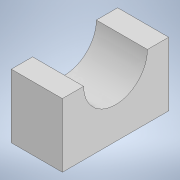
# Autodesk Inventor part: Top Part Ramp
Saved by Autodesk Inventor 2021 (Build 250183000, 183)
## iProperties
Created: 2021-03-30
Part Number: Top Part Ramp
Material: Generic
Document SubType Name: Modeling
Designer: Nabeel Azafer
Density: 1 g/cm^3
Appearance: Default
Author: Nabeel Azafer
Autodesk Inventor part; units mm, degrees
ref_plane "YZ Plane" through (0, 0, 0) normal (1, 0, 0) x (0, 1, 0)
ref_plane "XZ Plane" through (0, 0, 0) normal (0, 1, 0) x (-1, 0, 0)
ref_plane "XY Plane" through (0, 0, 0) normal (0, 0, 1) x (1, 0, 0)
sketch "Sketch1" plane through (0, 0, 0) normal (0, 0, 1) x (1, 0, 0)
  point P0 (0, 0)
sketch "Sketch2" plane through (0, 0, 0) normal (0, 0, 1) x (1, 0, 0)
  line L0 (0, 0) -> (12, 0)
  line L1 (12, 0) -> (12, 15)
  line L2 (12, 15) -> (0, 15)
  line L3 (0, 15) -> (0, 0)
  dimension "d0" = 12
  dimension "d1" = 15
  constraints: 8 end point, 2 parallel, 1 horizontal, 1 perpendicular
  measures "d0" distance of L0.start L0.end
  measures "d1" distance of L2.end L0.start
extrude "Extrusion1" add sketch "Sketch2" along normal blind 25
sketch "Sketch3" plane through (12, 0, 0) normal (1, 0, 0) x (0, 0, -1)
  line L0 (0, 15) -> (-25, 15) projected
  line L1 (0, 0) -> (-25, 0) projected
  line L2 (-25, 15) -> (-20, 15)
  line L3 (-20, 15) -> (-20, 0)
  line L4 (-20, 0) -> (-25, 0)
  line L5 (-25, 0) -> (-25, 15)
  line L6 (0, 0) -> (0, 15) projected
  line L7 (0, 15) -> (-5, 15)
  line L8 (-5, 15) -> (-5, 0)
  line L9 (-5, 0) -> (0, 0)
  line L10 (0, 0) -> (0, 15)
  arc A0 (-20, 15) -> (-5, 15) centre (-12.5, 15) ccw
  dimension "d4" = 5
  dimension "d5" = 5
  dimension "d6" = 7.5
  constraints: 16 end point, 4 parallel, 2 horizontal, 2 perpendicular, 2 point on circle, 2 point on line, 1 centre point
  measures "d4" distance of L3.end L4.end
  measures "d5" distance of L9.end L8.end
  measures "d6" radius of A0
extrude "Extrusion2" cut sketch "Sketch3" against normal blind 25 contours A0 L0
body "Solid1"
